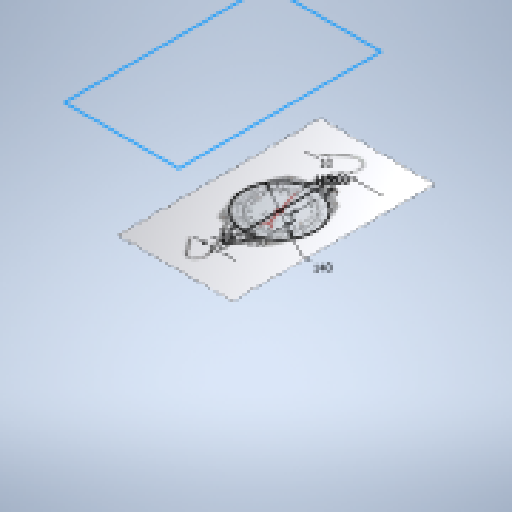
# Autodesk Inventor part: waage
Saved by Autodesk Inventor 2025 (Build 290162010, 162A)
## iProperties
Created: 2025-01-27
Part Number: waage
Material: Generisch
Document SubType Name: Modeling
Designer: Admin
Density: 1 g/cm^3
Appearance: Vorgabe
Author: Admin
Autodesk Inventor part; units mm, degrees
ref_plane "YZ Plane" through (0, 0, 0) normal (1, 0, 0) x (0, 1, 0)
ref_plane "XZ Plane" through (0, 0, 0) normal (0, 1, 0) x (-1, 0, 0)
ref_plane "XY Plane" through (0, 0, 0) normal (0, 0, 1) x (1, 0, 0)
sketch "Skizze2" plane through (0, 0, 0) normal (0, 0, 1) x (1, 0, 0)
  line L0 (-117.4666, 197.4366) -> (107.72, 197.4366) construction
  line L1 (107.72, 197.4366) -> (107.72, -200.7323) construction
  line L2 (107.72, -200.7323) -> (-117.4666, -200.7323) construction
  line L3 (-117.4666, -200.7323) -> (-117.4666, 197.4366) construction
  circle A0 centre (0, 0) radius 70
  line L4 (-20.6981, 66.87) -> (-5, 110)
  line L5 (-5, 110) -> (5, 110)
  line L6 (5, 110) -> (20.6981, 66.87)
  line L7 (-20.6981, -66.87) -> (-5, -110)
  line L8 (-5, -110) -> (5, -110)
  line L9 (5, -110) -> (20.6981, -66.87)
  line L10 (0, 110) -> (0, 0)
  line L11 (0, 0) -> (0, -110)
  dimension "d3" = 110
  dimension "d4" = 110
  dimension "d5" = 110
  dimension "d8" = 140
  dimension "d9" = 110
  dimension "d10" = 110
  dimension "d11" = 110
  dimension "d12" = 10
  dimension "d13" = 10
  constraints: 16 end point, 4 point on circle, 2 horizontal, 2 midpoint, 1 centre point, 1 collinear, 1 vertical, 5 other
  measures "d3" angle of L5 L4
  measures "d4" angle of L5 L6
  measures "d5" distance of L10.end L10.start
  measures "d8" diameter of A0
  measures "d9" distance from line of L8 L10.end
  measures "d10" angle of L8 L9
  measures "d11" angle of L8 L7
  measures "d12" distance of L4.end L5.end
  measures "d13" distance of L7.end L8.end
extrude "Extrusion1" add sketch "Skizze2" along normal blind 20 contours A0 L11 L10 | L10 L11 A0
extrude "Extrusion2" add sketch "Skizze2" along normal blind 7 contours A0 L10 L5 L6 | L9 L8 L11 A0 | A0 L4 L5 L10 | L11 L8 L7 A0
sketch "Skizze3" plane through (0, 0, 20) normal (0, 0, 1) x (1, 0, 0)
  line L0 (-65, 65) -> (65, 65) construction
  line L1 (65, 65) -> (65, -65.4377) construction
  line L2 (65, -65.4377) -> (-65, -65.4377) construction
  line L3 (-65, -65.4377) -> (-65, 65) construction
  point P0 (0, 0)
  constraints: 2 other
